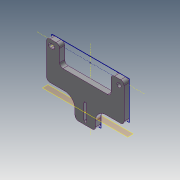
# Autodesk Inventor part: J005643
Saved by Autodesk Inventor 2015 SP1 (Build 190203100, 203)
## iProperties
Created: 2014-12-01
Material: Generic
Vendor: HHMI: JFRC - ID&F
Document SubType Name: Modeling
Designer: ARNOLDJ
Density: 1 g/cm^3
Appearance: Default
Description: BRACKET TO MOUNT TRACKING CAMERA
Part Number: J005643
RuleStatus: InUse
AfterDocSave0: file://Part Number Cleaner
DESIGN DEPARTMENT: HHMI: JFRC - ID&F
ALTERED ITEM PART NUMBER: N/A
ALTERED ITEM VENDOR: N/A
ALTERED ITEM DESCRIPTION: N/A
Revision Number: 0
Autodesk Inventor part; units mm, degrees
sketch "Sketch1" plane through (0, 0, 0) normal (0, 0, 1) x (1, 0, 0)
  line L0 (-100.457, 0) -> (100.457, 0) construction
  line L1 (0, 31.242) -> (0, -116.332) construction
  circle A0 centre (-62.4459, 0) radius 3.8354 construction
  circle A1 centre (62.4459, 0) radius 3.8354 construction
  line L2 (-62.4459, 0) -> (62.4459, 0) construction
  line L3 (-71.755, 10.16) -> (71.755, 10.16)
  line L4 (71.755, 10.16) -> (71.755, -59.69)
  line L5 (19.05, -95.25) -> (-19.05, -95.25)
  line L6 (-71.755, -59.69) -> (-71.755, 10.16)
  circle A2 centre (-64.3509, 0) radius 3.8354
  circle A3 centre (-60.5409, 0) radius 3.8354
  line L7 (-64.3559, 3.8354) -> (-60.5409, 3.8354)
  line L8 (-64.3763, -3.8353) -> (-60.541, -3.8354)
  circle A4 centre (62.4459, 0) radius 3.8354
  line L9 (-71.755, -59.69) -> (-57.1821, -59.69)
  line L10 (53.5114, -59.69) -> (71.755, -59.69)
  line L11 (-19.05, -95.25) -> (-19.05, -59.69)
  line L12 (-19.05, -59.69) -> (-57.1821, -59.69)
  line L13 (19.05, -95.25) -> (19.05, -59.69)
  line L14 (19.05, -59.69) -> (53.5114, -59.69)
  point P0 (0, 0)
  point P1 (0, 0)
  point P2 (0, 10.16)
  point P3 (0, -95.25)
  dimension "d0" = 7.6708
  dimension "d1" = 124.8918
  dimension "d2" = 143.51
  dimension "d3" = 10.16
  dimension "d7" = 38.1
  dimension "d16" = 7.6708
  dimension "d17" = 1.905
  dimension "d18" = 1.905
  dimension "d29" = 95.25
  dimension "d31" = 59.69
  constraints: 26 end point, 5 centre point, 5 horizontal, 4 equal radius, 4 point on circle, 4 point on line, 3 coincident, 3 midpoint, 2 horizontal alignment, 2 parallel, 2 tangent, 2 vertical, 2 vertical alignment, 1 perpendicular
  measures "d0" diameter of A0
  measures "d1" distance of L2.end L2.start
  measures "d2" distance of L3.start L3.end
  measures "d3" distance from line of L3 point (0, 0)
  measures "d7" distance of L5.start L5.end
  measures "d16" diameter of A1
  measures "d17" distance of L2.start A2.centre
  measures "d18" distance of L2.start A3.centre
  measures "d29" distance from line of point (0, 0) L5
  measures "d31" distance from line of L12 point (0, 0)
ref_plane "Work Plane1" through (0, -74.9046, 0) normal (0, 1, 0) x (-1, 0, 0)
extrude "Extrusion1" add sketch "Sketch1" along normal blind 9.525 contours L3 L4 L10 L14 L13 L5 L11 L12 L9 L6 | A2 A3 L8 | A2 A3 | L7 A3 A2 | A3 A2 | A2 A3 | A4
sketch "Sketch2" plane through (0, 0, 9.525) normal (0, 0, 1) x (1, 0, 0)
  line L0 (-2.3812, -58.3946) -> (2.3813, -58.3946)
  line L1 (2.3813, -58.3946) -> (2.3812, -91.4146)
  line L2 (2.3812, -91.4146) -> (-2.3812, -91.4146)
  line L3 (-2.3812, -91.4146) -> (-2.3812, -58.3946)
  line L4 (-2.3813, -74.9046) -> (2.3813, -74.9046) construction
  line L5 (-100.457, -74.9046) -> (100.457, -74.9046) projected
  point P0 (0, 0)
  point P1 (0, -58.3946)
  dimension "d10" = 4.7625
  dimension "d11" = 33.02
  dimension "d12" = 74.9046
  dimension "d28" = 0
  constraints: 10 end point, 3 midpoint, 2 parallel, 1 horizontal, 1 perpendicular, 1 vertical alignment
  measures "d10" distance of L0.start L0.end
  measures "d11" distance of L2.end L0.start
  measures "d12" distance from line of L4 point (0, 0)
  measures "d28" distance between parallel lines of L5 L4
extrude "Extrusion2" cut sketch "Sketch2" against normal up to next
fillet "Fillet1" radius 2.3813 4 edges at (-2.3812, -58.3946, 4.7625) (2.3813, -58.3946, 4.7625) (2.3812, -91.4146, 4.7625) (-2.3812, -91.4146, 4.7625)
extrude "Extrusion3" cut sketch "Sketch1" along normal blind 9.525 contours A2 A3 L8 | A2 A3 | L7 A3 A2 | A3 A2 | A2 A3 | A4
sketch "Sketch4" plane through (0, 0, 0) normal (0, 0, 1) x (1, 0, 0)
  line L0 (-71.755, 10.16) -> (71.755, 10.16) projected
  line L1 (-47.625, 10.16) -> (47.625, 10.16)
  line L2 (47.625, 10.16) -> (47.625, -25.4)
  line L3 (47.625, -25.4) -> (-47.625, -25.4)
  line L4 (-47.625, -25.4) -> (-47.625, 10.16)
  line L5 (0, -25.4) -> (0, 10.16) construction
  point P0 (0, 0)
  dimension "d21" = 35.56
  dimension "d22" = 95.25
  dimension "d23" = 0
  constraints: 10 end point, 2 midpoint, 2 parallel, 1 horizontal, 1 perpendicular, 1 point on line
  measures "d21" distance of L3.end L1.start
  measures "d22" distance of L2.end L3.end
  measures "d23" horizontal distance of L5.start point (0, 0)
extrude "Extrusion4" cut sketch "Sketch4" along normal up to next
fillet "Fillet2" radius 6.35 10 edges at (-47.625, -25.4, 4.7625) (-47.625, 10.16, 4.7625) (-71.755, 10.16, 4.7625) (47.625, -25.4, 4.7625) (47.625, 10.16, 4.7625) (71.755, 10.16, 4.7625) (71.755, -59.69, 4.7625) (-71.755, -59.69, 4.7625) (19.05, -95.25, 4.7625) (-19.05, -95.25, 4.7625)
fillet "Fillet3" radius 19.05 2 edges at (19.05, -59.69, 4.7625) (-19.05, -59.69, 4.7625)
body "Solid1"
